Autodesk Fusion 360 part; units mm, degrees
(part 15 of 18)
  arc A2317 (195.6454, -39.5852) -> (195.5255, -39.5852) centre (195.5855, -39.5852) ccw
  arc A2318 (195.5255, -77.7107) -> (195.6454, -77.7107) centre (195.5855, -77.7107) ccw
  arc A2319 (195.6454, -77.7107) -> (195.5255, -77.7107) centre (195.5855, -77.7107) ccw
  arc A2320 (195.5255, -58.648) -> (195.6454, -58.648) centre (195.5855, -58.648) ccw
  arc A2321 (195.6454, -58.648) -> (195.5255, -58.648) centre (195.5855, -58.648) ccw
  arc A2322 (195.6454, -20.5352) -> (195.5255, -20.5352) centre (195.5855, -20.5352) ccw
  arc A2323 (195.5255, -20.5352) -> (195.6454, -20.5352) centre (195.5855, -20.5352) ccw
  arc A2324 (203.2985, -3.41) -> (203.1785, -3.41) centre (203.2385, -3.41) ccw
  arc A2325 (203.1785, -3.41) -> (203.2985, -3.41) centre (203.2385, -3.41) ccw
  arc A2326 (201.3935, -6.331) -> (201.2735, -6.331) centre (201.3335, -6.331) ccw
  arc A2327 (201.2735, -6.331) -> (201.3935, -6.331) centre (201.3335, -6.331) ccw
  arc A2328 (204.8803, -5.2261) -> (205.0003, -5.2261) centre (204.9403, -5.2261) ccw
  arc A2329 (205.0003, -5.2261) -> (204.8803, -5.2261) centre (204.9403, -5.2261) ccw
  arc A2330 (-5.7971, 1.189) -> (-5.6771, 1.189) centre (-5.7371, 1.189) ccw
  arc A2331 (-5.6771, 1.189) -> (-5.7971, 1.189) centre (-5.7371, 1.189) ccw
  arc A2332 (195.2538, -3.4209) -> (195.1338, -3.4209) centre (195.1938, -3.4209) ccw
  arc A2333 (195.1338, -3.4209) -> (195.2538, -3.4209) centre (195.1938, -3.4209) ccw
  arc A2334 (172.1523, -5.568) -> (172.2723, -5.568) centre (172.2123, -5.568) ccw
  arc A2335 (172.2723, -5.568) -> (172.1523, -5.568) centre (172.2123, -5.568) ccw
  arc A2336 (201.4005, -1.505) -> (201.5205, -1.505) centre (201.4605, -1.505) ccw
  arc A2337 (201.5205, -1.505) -> (201.4005, -1.505) centre (201.4605, -1.505) ccw
  arc A2338 (207.5145, -5.263) -> (207.6344, -5.263) centre (207.5744, -5.263) ccw
  arc A2339 (207.6344, -5.263) -> (207.5145, -5.263) centre (207.5744, -5.263) ccw
  arc A2340 (186.8463, -7.1311) -> (186.9662, -7.1311) centre (186.9063, -7.1311) ccw
  arc A2341 (186.9662, -7.1311) -> (186.8463, -7.1311) centre (186.9063, -7.1311) ccw
  arc A2342 (183.8745, -6.331) -> (183.9944, -6.331) centre (183.9345, -6.331) ccw
  arc A2343 (183.9944, -6.331) -> (183.8745, -6.331) centre (183.9345, -6.331) ccw
  arc A2344 (212.5755, -3.786) -> (212.6955, -3.786) centre (212.6355, -3.786) ccw
  arc A2345 (212.6955, -3.786) -> (212.5755, -3.786) centre (212.6355, -3.786) ccw
  arc A2346 (138.4953, -77.7107) -> (138.3754, -77.7107) centre (138.4354, -77.7107) ccw
  arc A2347 (138.3754, -77.7107) -> (138.4953, -77.7107) centre (138.4354, -77.7107) ccw
  arc A2348 (138.3754, -20.5352) -> (138.4953, -20.5352) centre (138.4354, -20.5352) ccw
  arc A2349 (138.4953, -20.5352) -> (138.3754, -20.5352) centre (138.4354, -20.5352) ccw
  arc A2350 (138.3754, -39.5852) -> (138.4953, -39.5852) centre (138.4354, -39.5852) ccw
  arc A2351 (138.4953, -39.5852) -> (138.3754, -39.5852) centre (138.4354, -39.5852) ccw
  arc A2352 (138.4953, -58.648) -> (138.3754, -58.648) centre (138.4354, -58.648) ccw
  arc A2353 (138.3754, -58.648) -> (138.4953, -58.648) centre (138.4354, -58.648) ccw
  arc A2354 (157.5454, -20.5352) -> (157.4254, -20.5352) centre (157.4854, -20.5352) ccw
  arc A2355 (157.4254, -20.5352) -> (157.5454, -20.5352) centre (157.4854, -20.5352) ccw
  arc A2356 (157.5454, -77.7107) -> (157.4254, -77.7107) centre (157.4854, -77.7107) ccw
  arc A2357 (157.4254, -77.7107) -> (157.5454, -77.7107) centre (157.4854, -77.7107) ccw
  arc A2358 (157.4254, -58.648) -> (157.5454, -58.648) centre (157.4854, -58.648) ccw
  arc A2359 (157.5454, -58.648) -> (157.4254, -58.648) centre (157.4854, -58.648) ccw
  arc A2360 (157.4254, -39.5852) -> (157.5454, -39.5852) centre (157.4854, -39.5852) ccw
  arc A2361 (157.5454, -39.5852) -> (157.4254, -39.5852) centre (157.4854, -39.5852) ccw
  arc A2362 (176.4755, -20.5352) -> (176.5954, -20.5352) centre (176.5354, -20.5352) ccw
  arc A2363 (176.5954, -20.5352) -> (176.4755, -20.5352) centre (176.5354, -20.5352) ccw
  arc A2364 (176.5954, -77.7107) -> (176.4755, -77.7107) centre (176.5354, -77.7107) ccw
  arc A2365 (176.4755, -77.7107) -> (176.5954, -77.7107) centre (176.5354, -77.7107) ccw
  arc A2366 (176.4755, -58.648) -> (176.5954, -58.648) centre (176.5354, -58.648) ccw
  arc A2367 (176.5954, -58.648) -> (176.4755, -58.648) centre (176.5354, -58.648) ccw
  arc A2368 (176.4755, -39.5852) -> (176.5954, -39.5852) centre (176.5354, -39.5852) ccw
  arc A2369 (176.5954, -39.5852) -> (176.4755, -39.5852) centre (176.5354, -39.5852) ccw
  arc A2370 (100.3953, -77.7107) -> (100.2753, -77.7107) centre (100.3353, -77.7107) ccw
  arc A2371 (100.2753, -77.7107) -> (100.3953, -77.7107) centre (100.3353, -77.7107) ccw
  arc A2372 (100.3953, -58.648) -> (100.2753, -58.648) centre (100.3353, -58.648) ccw
  arc A2373 (100.2753, -58.648) -> (100.3953, -58.648) centre (100.3353, -58.648) ccw
  arc A2374 (100.3953, -20.5352) -> (100.2753, -20.5352) centre (100.3353, -20.5352) ccw
  arc A2375 (100.2753, -20.5352) -> (100.3953, -20.5352) centre (100.3353, -20.5352) ccw
  arc A2376 (100.3953, -39.5852) -> (100.2753, -39.5852) centre (100.3353, -39.5852) ccw
  arc A2377 (100.2753, -39.5852) -> (100.3953, -39.5852) centre (100.3353, -39.5852) ccw
  arc A2378 (119.4453, -20.5352) -> (119.3253, -20.5352) centre (119.3853, -20.5352) ccw
  arc A2379 (119.3253, -20.5352) -> (119.4453, -20.5352) centre (119.3853, -20.5352) ccw
  arc A2380 (119.3253, -58.648) -> (119.4453, -58.648) centre (119.3853, -58.648) ccw
  arc A2381 (119.4453, -58.648) -> (119.3253, -58.648) centre (119.3853, -58.648) ccw
  arc A2382 (119.3253, -39.5852) -> (119.4453, -39.5852) centre (119.3853, -39.5852) ccw
  arc A2383 (119.4453, -39.5852) -> (119.3253, -39.5852) centre (119.3853, -39.5852) ccw
  arc A2384 (119.3253, -77.7107) -> (119.4453, -77.7107) centre (119.3853, -77.7107) ccw
  arc A2385 (119.4453, -77.7107) -> (119.3253, -77.7107) centre (119.3853, -77.7107) ccw
  arc A2386 (5.0251, -77.7107) -> (5.1451, -77.7107) centre (5.0851, -77.7107) ccw
  arc A2387 (5.1451, -77.7107) -> (5.0251, -77.7107) centre (5.0851, -77.7107) ccw
  arc A2388 (24.0752, -77.7107) -> (24.1951, -77.7107) centre (24.1351, -77.7107) ccw
  arc A2389 (24.1951, -77.7107) -> (24.0752, -77.7107) centre (24.1351, -77.7107) ccw
  arc A2390 (43.1252, -77.7107) -> (43.2451, -77.7107) centre (43.1852, -77.7107) ccw
  arc A2391 (43.2451, -77.7107) -> (43.1252, -77.7107) centre (43.1852, -77.7107) ccw
  arc A2392 (62.2952, -20.5352) -> (62.1752, -20.5352) centre (62.2352, -20.5352) ccw
  arc A2393 (62.1752, -20.5352) -> (62.2952, -20.5352) centre (62.2352, -20.5352) ccw
  arc A2394 (62.1752, -77.7107) -> (62.2952, -77.7107) centre (62.2352, -77.7107) ccw
  arc A2395 (62.2952, -77.7107) -> (62.1752, -77.7107) centre (62.2352, -77.7107) ccw
  arc A2396 (62.1752, -39.5852) -> (62.2952, -39.5852) centre (62.2352, -39.5852) ccw
  arc A2397 (62.2952, -39.5852) -> (62.1752, -39.5852) centre (62.2352, -39.5852) ccw
  arc A2398 (62.1752, -58.648) -> (62.2952, -58.648) centre (62.2352, -58.648) ccw
  arc A2399 (62.2952, -58.648) -> (62.1752, -58.648) centre (62.2352, -58.648) ccw
  arc A2400 (81.2253, -39.5852) -> (81.3452, -39.5852) centre (81.2852, -39.5852) ccw
  arc A2401 (81.3452, -39.5852) -> (81.2253, -39.5852) centre (81.2852, -39.5852) ccw
  arc A2402 (81.2253, -77.7107) -> (81.3452, -77.7107) centre (81.2852, -77.7107) ccw
  arc A2403 (81.3452, -77.7107) -> (81.2253, -77.7107) centre (81.2852, -77.7107) ccw
  arc A2404 (81.2253, -20.5352) -> (81.3452, -20.5352) centre (81.2852, -20.5352) ccw
  arc A2405 (81.3452, -20.5352) -> (81.2253, -20.5352) centre (81.2852, -20.5352) ccw
  arc A2406 (81.3452, -58.648) -> (81.2253, -58.648) centre (81.2852, -58.648) ccw
  arc A2407 (81.2253, -58.648) -> (81.3452, -58.648) centre (81.2852, -58.648) ccw
  arc A2408 (5.0251, -58.648) -> (5.1451, -58.648) centre (5.0851, -58.648) ccw
  arc A2409 (5.1451, -58.648) -> (5.0251, -58.648) centre (5.0851, -58.648) ccw
  arc A2410 (5.0251, -20.5352) -> (5.1451, -20.5352) centre (5.0851, -20.5352) ccw
  arc A2411 (5.1451, -20.5352) -> (5.0251, -20.5352) centre (5.0851, -20.5352) ccw
  arc A2412 (5.1451, -39.5852) -> (5.0251, -39.5852) centre (5.0851, -39.5852) ccw
  arc A2413 (5.0251, -39.5852) -> (5.1451, -39.5852) centre (5.0851, -39.5852) ccw
  arc A2414 (24.0752, -39.5852) -> (24.1951, -39.5852) centre (24.1351, -39.5852) ccw
  arc A2415 (24.1951, -39.5852) -> (24.0752, -39.5852) centre (24.1351, -39.5852) ccw
  arc A2416 (24.0752, -20.5352) -> (24.1951, -20.5352) centre (24.1351, -20.5352) ccw
  arc A2417 (24.1951, -20.5352) -> (24.0752, -20.5352) centre (24.1351, -20.5352) ccw
  arc A2418 (24.0752, -58.648) -> (24.1951, -58.648) centre (24.1351, -58.648) ccw
  arc A2419 (24.1951, -58.648) -> (24.0752, -58.648) centre (24.1351, -58.648) ccw
  arc A2420 (43.1252, -20.5352) -> (43.2451, -20.5352) centre (43.1852, -20.5352) ccw
  arc A2421 (43.2451, -20.5352) -> (43.1252, -20.5352) centre (43.1852, -20.5352) ccw
  arc A2422 (43.1252, -58.648) -> (43.2451, -58.648) centre (43.1852, -58.648) ccw
  arc A2423 (43.2451, -58.648) -> (43.1252, -58.648) centre (43.1852, -58.648) ccw
  arc A2424 (43.2451, -39.5852) -> (43.1252, -39.5852) centre (43.1852, -39.5852) ccw
  arc A2425 (43.1252, -39.5852) -> (43.2451, -39.5852) centre (43.1852, -39.5852) ccw
  arc A2426 (214.6955, -20.5352) -> (214.5755, -20.5352) centre (214.6355, -20.5352) ccw
  arc A2427 (214.5755, -20.5352) -> (214.6955, -20.5352) centre (214.6355, -20.5352) ccw
  arc A2428 (214.6955, -77.7107) -> (214.5755, -77.7107) centre (214.6355, -77.7107) ccw
  arc A2429 (214.5755, -77.7107) -> (214.6955, -77.7107) centre (214.6355, -77.7107) ccw
  arc A2430 (214.5755, -58.648) -> (214.6955, -58.648) centre (214.6355, -58.648) ccw
  arc A2431 (214.6955, -58.648) -> (214.5755, -58.648) centre (214.6355, -58.648) ccw
  arc A2432 (214.6955, -39.5852) -> (214.5755, -39.5852) centre (214.6355, -39.5852) ccw
  arc A2433 (214.5755, -39.5852) -> (214.6955, -39.5852) centre (214.6355, -39.5852) ccw
  arc A2434 (195.5255, -39.5852) -> (195.6454, -39.5852) centre (195.5855, -39.5852) ccw
  arc A2435 (195.6454, -39.5852) -> (195.5255, -39.5852) centre (195.5855, -39.5852) ccw
  arc A2436 (195.6454, -77.7107) -> (195.5255, -77.7107) centre (195.5855, -77.7107) ccw
  arc A2437 (195.5255, -77.7107) -> (195.6454, -77.7107) centre (195.5855, -77.7107) ccw
  arc A2438 (195.6454, -58.648) -> (195.5255, -58.648) centre (195.5855, -58.648) ccw
  arc A2439 (195.5255, -58.648) -> (195.6454, -58.648) centre (195.5855, -58.648) ccw
  arc A2440 (195.5255, -20.5352) -> (195.6454, -20.5352) centre (195.5855, -20.5352) ccw
  arc A2441 (195.6454, -20.5352) -> (195.5255, -20.5352) centre (195.5855, -20.5352) ccw
  arc A2442 (203.2985, -3.41) -> (203.1785, -3.41) centre (203.2385, -3.41) ccw
  arc A2443 (203.1785, -3.41) -> (203.2985, -3.41) centre (203.2385, -3.41) ccw
  arc A2444 (201.3935, -6.331) -> (201.2735, -6.331) centre (201.3335, -6.331) ccw
  arc A2445 (201.2735, -6.331) -> (201.3935, -6.331) centre (201.3335, -6.331) ccw
  arc A2446 (205.0003, -5.2261) -> (204.8803, -5.2261) centre (204.9403, -5.2261) ccw
  arc A2447 (204.8803, -5.2261) -> (205.0003, -5.2261) centre (204.9403, -5.2261) ccw
  arc A2448 (-5.6771, 1.189) -> (-5.7971, 1.189) centre (-5.7371, 1.189) ccw
  arc A2449 (-5.7971, 1.189) -> (-5.6771, 1.189) centre (-5.7371, 1.189) ccw
  arc A2450 (195.2538, -3.4209) -> (195.1338, -3.4209) centre (195.1938, -3.4209) ccw
  arc A2451 (195.1338, -3.4209) -> (195.2538, -3.4209) centre (195.1938, -3.4209) ccw
  arc A2452 (172.1523, -5.568) -> (172.2723, -5.568) centre (172.2123, -5.568) ccw
  arc A2453 (172.2723, -5.568) -> (172.1523, -5.568) centre (172.2123, -5.568) ccw
  arc A2454 (10.2131, -8.0011) -> (9.1131, -8.0011) centre (9.6631, -8.0011) ccw
  arc A2455 (9.1131, -8.0011) -> (10.2131, -8.0011) centre (9.6631, -8.0011) ccw
  arc A2456 (10.2131, -5.4611) -> (9.1131, -5.4611) centre (9.6631, -5.4611) ccw
  arc A2457 (9.1131, -5.4611) -> (10.2131, -5.4611) centre (9.6631, -5.4611) ccw
  arc A2458 (10.2131, -2.9211) -> (9.1131, -2.9211) centre (9.6631, -2.9211) ccw
  arc A2459 (9.1131, -2.9211) -> (10.2131, -2.9211) centre (9.6631, -2.9211) ccw
  arc A2460 (-5.3871, -8.0011) -> (-4.287, -8.0011) centre (-4.8371, -8.0011) ccw
  arc A2461 (-4.287, -8.0011) -> (-5.3871, -8.0011) centre (-4.8371, -8.0011) ccw
  arc A2462 (-4.287, -2.9211) -> (-5.3871, -2.9211) centre (-4.8371, -2.9211) ccw
  arc A2463 (-5.3871, -2.9211) -> (-4.287, -2.9211) centre (-4.8371, -2.9211) ccw
  arc A2464 (175.5224, -4.318) -> (176.5223, -4.318) centre (176.0224, -4.318) ccw
  arc A2465 (176.5223, -4.318) -> (175.5224, -4.318) centre (176.0224, -4.318) ccw
  arc A2466 (173.9823, -4.318) -> (172.9824, -4.318) centre (173.4823, -4.318) ccw
  arc A2467 (172.9824, -4.318) -> (173.9823, -4.318) centre (173.4823, -4.318) ccw
  line L8932 (201.4604, -1.505) -> (201.4604, -2.305)
  line L8933 (201.4604, -2.305) -> (201.1604, -2.305)
  line L8934 (201.1604, -1.505) -> (201.4604, -1.505)
  line L8935 (201.1604, -2.305) -> (201.1604, -1.505)
  line L8936 (199.8604, -1.505) -> (199.8604, -2.305)
  line L8937 (200.1604, -2.305) -> (200.1604, -1.505)
  line L8938 (199.8604, -2.305) -> (200.1604, -2.305)
  line L8939 (200.1604, -1.505) -> (199.8604, -1.505)
  line L8940 (207.5745, -6.0629) -> (207.9745, -6.0629)
  line L8941 (207.9745, -6.2629) -> (207.5745, -6.2629)
  line L8942 (207.5745, -6.2629) -> (207.5745, -6.0629)
  line L8943 (207.9745, -6.0629) -> (207.9745, -6.2629)
  line L8944 (207.9745, -6.6629) -> (207.5745, -6.6629)
  line L8945 (207.9745, -6.4629) -> (207.9745, -6.6629)
  line L8946 (207.5745, -6.6629) -> (207.5745, -6.4629)
  line L8947 (207.5745, -6.4629) -> (207.9745, -6.4629)
  line L8948 (207.9745, -7.0629) -> (207.5745, -7.0629)
  line L8949 (207.9745, -6.8629) -> (207.9745, -7.0629)
  line L8950 (207.5745, -7.0629) -> (207.5745, -6.8629)
  line L8951 (207.5745, -6.8629) -> (207.9745, -6.8629)
  line L8952 (207.9745, -7.4629) -> (207.5745, -7.4629)
  line L8953 (207.5745, -7.2629) -> (207.9745, -7.2629)
  line L8954 (207.5745, -7.4629) -> (207.5745, -7.2629)
  line L8955 (207.9745, -7.2629) -> (207.9745, -7.4629)
  line L8956 (207.5745, -7.6629) -> (207.9745, -7.6629)
  line L8957 (207.9745, -7.6629) -> (207.9745, -7.8629)
  line L8958 (207.5745, -7.8629) -> (207.5745, -7.6629)
  line L8959 (207.9745, -7.8629) -> (207.5745, -7.8629)
  line L8960 (207.5745, -8.0629) -> (207.9745, -8.0629)
  line L8961 (207.9745, -8.2629) -> (207.5745, -8.2629)
  line L8962 (207.9745, -8.0629) -> (207.9745, -8.2629)
  line L8963 (207.5745, -8.2629) -> (207.5745, -8.0629)
  line L8964 (207.9745, -8.4629) -> (207.9745, -8.6629)
  line L8965 (207.5745, -8.4629) -> (207.9745, -8.4629)
  line L8966 (207.9745, -8.6629) -> (207.5745, -8.6629)
  line L8967 (207.5745, -8.6629) -> (207.5745, -8.4629)
  line L8968 (207.5745, -9.0629) -> (207.5745, -8.8629)
  line L8969 (207.9745, -8.8629) -> (207.9745, -9.0629)
  line L8970 (207.5745, -8.8629) -> (207.9745, -8.8629)
  line L8971 (207.9745, -9.0629) -> (207.5745, -9.0629)
  line L8972 (207.9745, -9.2629) -> (207.9745, -9.4629)
  line L8973 (207.5745, -9.2629) -> (207.9745, -9.2629)
  line L8974 (207.5745, -9.4629) -> (207.5745, -9.2629)
  line L8975 (207.9745, -9.4629) -> (207.5745, -9.4629)
  line L8976 (207.9745, -9.6629) -> (207.9745, -9.8629)
  line L8977 (207.5745, -9.8629) -> (207.5745, -9.6629)
  line L8978 (207.9745, -9.8629) -> (207.5745, -9.8629)
  line L8979 (207.5745, -9.6629) -> (207.9745, -9.6629)
  line L8980 (207.5745, -10.2629) -> (207.5745, -10.0629)
  line L8981 (207.5745, -10.0629) -> (207.9745, -10.0629)
  line L8982 (207.9745, -10.2629) -> (207.5745, -10.2629)
  line L8983 (207.9745, -10.0629) -> (207.9745, -10.2629)
  line L8984 (207.5745, -10.6629) -> (207.5745, -10.4629)
  line L8985 (207.9745, -10.4629) -> (207.9745, -10.6629)
  line L8986 (207.9745, -10.6629) -> (207.5745, -10.6629)
  line L8987 (207.5745, -10.4629) -> (207.9745, -10.4629)
  line L8988 (207.9745, -11.0629) -> (207.5745, -11.0629)
  line L8989 (207.5745, -10.8629) -> (207.9745, -10.8629)
  line L8990 (207.9745, -10.8629) -> (207.9745, -11.0629)
  line L8991 (207.5745, -11.0629) -> (207.5745, -10.8629)
  line L8992 (207.9745, -11.4629) -> (207.5745, -11.4629)
  line L8993 (207.5745, -11.4629) -> (207.5745, -11.2629)
  line L8994 (207.9745, -11.2629) -> (207.9745, -11.4629)
  line L8995 (207.5745, -11.2629) -> (207.9745, -11.2629)
  line L8996 (208.5745, -12.2629) -> (208.3745, -12.2629)
  line L8997 (208.3745, -11.8629) -> (208.5745, -11.8629)
  line L8998 (208.3745, -12.2629) -> (208.3745, -11.8629)
  line L8999 (208.5745, -11.8629) -> (208.5745, -12.2629)
  line L9000 (208.9745, -12.2629) -> (208.7745, -12.2629)
  line L9001 (208.9745, -11.8629) -> (208.9745, -12.2629)
  line L9002 (208.7745, -11.8629) -> (208.9745, -11.8629)
  line L9003 (208.7745, -12.2629) -> (208.7745, -11.8629)
  line L9004 (209.1745, -11.8629) -> (209.3745, -11.8629)
  line L9005 (209.3745, -12.2629) -> (209.1745, -12.2629)
  line L9006 (209.1745, -12.2629) -> (209.1745, -11.8629)
  line L9007 (209.3745, -11.8629) -> (209.3745, -12.2629)
  line L9008 (209.5745, -11.8629) -> (209.7745, -11.8629)
  line L9009 (209.7745, -12.2629) -> (209.5745, -12.2629)
  line L9010 (209.7745, -11.8629) -> (209.7745, -12.2629)
  line L9011 (209.5745, -12.2629) -> (209.5745, -11.8629)
  line L9012 (210.1745, -12.2629) -> (209.9745, -12.2629)
  line L9013 (209.9745, -12.2629) -> (209.9745, -11.8629)
  line L9014 (209.9745, -11.8629) -> (210.1745, -11.8629)
  line L9015 (210.1745, -11.8629) -> (210.1745, -12.2629)
  line L9016 (210.3745, -12.2629) -> (210.3745, -11.8629)
  line L9017 (210.5745, -11.8629) -> (210.5745, -12.2629)
  line L9018 (210.5745, -12.2629) -> (210.3745, -12.2629)
  line L9019 (210.3745, -11.8629) -> (210.5745, -11.8629)
  line L9020 (210.7745, -12.2629) -> (210.7745, -11.8629)
  line L9021 (210.9745, -11.8629) -> (210.9745, -12.2629)
  line L9022 (210.7745, -11.8629) -> (210.9745, -11.8629)
  line L9023 (210.9745, -12.2629) -> (210.7745, -12.2629)
  line L9024 (211.3745, -12.2629) -> (211.1745, -12.2629)
  line L9025 (211.1745, -12.2629) -> (211.1745, -11.8629)
  line L9026 (211.3745, -11.8629) -> (211.3745, -12.2629)
  line L9027 (211.1745, -11.8629) -> (211.3745, -11.8629)
  line L9028 (211.7745, -11.8629) -> (211.7745, -12.2629)
  line L9029 (211.5745, -12.2629) -> (211.5745, -11.8629)
  line L9030 (211.7745, -12.2629) -> (211.5745, -12.2629)
  line L9031 (211.5745, -11.8629) -> (211.7745, -11.8629)
  line L9032 (211.9745, -11.8629) -> (212.1745, -11.8629)
  line L9033 (212.1745, -11.8629) -> (212.1745, -12.2629)
  line L9034 (212.1745, -12.2629) -> (211.9745, -12.2629)
  line L9035 (211.9745, -12.2629) -> (211.9745, -11.8629)
  line L9036 (212.3745, -12.2629) -> (212.3745, -11.8629)
  line L9037 (212.5745, -12.2629) -> (212.3745, -12.2629)
  line L9038 (212.3745, -11.8629) -> (212.5745, -11.8629)
  line L9039 (212.5745, -11.8629) -> (212.5745, -12.2629)
  line L9040 (212.7745, -11.8629) -> (212.9745, -11.8629)
  line L9041 (212.7745, -12.2629) -> (212.7745, -11.8629)
  line L9042 (212.9745, -11.8629) -> (212.9745, -12.2629)
  line L9043 (212.9745, -12.2629) -> (212.7745, -12.2629)
  line L9044 (213.3745, -11.8629) -> (213.3745, -12.2629)
  line L9045 (213.1745, -12.2629) -> (213.1745, -11.8629)
  line L9046 (213.3745, -12.2629) -> (213.1745, -12.2629)
  line L9047 (213.1745, -11.8629) -> (213.3745, -11.8629)
  line L9048 (213.7745, -12.2629) -> (213.5745, -12.2629)
  line L9049 (213.5745, -11.8629) -> (213.7745, -11.8629)
  line L9050 (213.5745, -12.2629) -> (213.5745, -11.8629)
  line L9051 (213.7745, -11.8629) -> (213.7745, -12.2629)
  line L9052 (214.5745, -11.4629) -> (214.5745, -11.2629)
  line L9053 (214.1745, -11.2629) -> (214.1745, -11.4629)
  line L9054 (214.5745, -11.2629) -> (214.1745, -11.2629)
  line L9055 (214.1745, -11.4629) -> (214.5745, -11.4629)
  line L9056 (214.5745, -11.0629) -> (214.5745, -10.8629)
  line L9057 (214.1745, -10.8629) -> (214.1745, -11.0629)
  line L9058 (214.5745, -10.8629) -> (214.1745, -10.8629)
  line L9059 (214.1745, -11.0629) -> (214.5745, -11.0629)
  line L9060 (214.1745, -10.6629) -> (214.5745, -10.6629)
  line L9061 (214.5745, -10.6629) -> (214.5745, -10.4629)
  line L9062 (214.1745, -10.4629) -> (214.1745, -10.6629)
  line L9063 (214.5745, -10.4629) -> (214.1745, -10.4629)
  line L9064 (214.5745, -10.2629) -> (214.5745, -10.0629)
  line L9065 (214.1745, -10.2629) -> (214.5745, -10.2629)
  line L9066 (214.5745, -10.0629) -> (214.1745, -10.0629)
  line L9067 (214.1745, -10.0629) -> (214.1745, -10.2629)
  line L9068 (214.1745, -9.8629) -> (214.5745, -9.8629)
  line L9069 (214.5745, -9.6629) -> (214.1745, -9.6629)
  line L9070 (214.5745, -9.8629) -> (214.5745, -9.6629)
  line L9071 (214.1745, -9.6629) -> (214.1745, -9.8629)
  line L9072 (214.5745, -9.4629) -> (214.5745, -9.2629)
  line L9073 (214.1745, -9.2629) -> (214.1745, -9.4629)
  line L9074 (214.1745, -9.4629) -> (214.5745, -9.4629)
  line L9075 (214.5745, -9.2629) -> (214.1745, -9.2629)
  line L9076 (214.5745, -9.0629) -> (214.5745, -8.8629)
  line L9077 (214.1745, -8.8629) -> (214.1745, -9.0629)
  line L9078 (214.1745, -9.0629) -> (214.5745, -9.0629)
  line L9079 (214.5745, -8.8629) -> (214.1745, -8.8629)
  line L9080 (214.1745, -8.4629) -> (214.1745, -8.6629)
  line L9081 (214.5745, -8.4629) -> (214.1745, -8.4629)
  line L9082 (214.5745, -8.6629) -> (214.5745, -8.4629)
  line L9083 (214.1745, -8.6629) -> (214.5745, -8.6629)
  line L9084 (214.1745, -8.2629) -> (214.5745, -8.2629)
  line L9085 (214.1745, -8.0629) -> (214.1745, -8.2629)
  line L9086 (214.5745, -8.2629) -> (214.5745, -8.0629)
  line L9087 (214.5745, -8.0629) -> (214.1745, -8.0629)
  line L9088 (214.1745, -7.8629) -> (214.5745, -7.8629)
  line L9089 (214.5745, -7.6629) -> (214.1745, -7.6629)
  line L9090 (214.1745, -7.6629) -> (214.1745, -7.8629)
  line L9091 (214.5745, -7.8629) -> (214.5745, -7.6629)
  line L9092 (214.5745, -7.4629) -> (214.5745, -7.2629)
  line L9093 (214.5745, -7.2629) -> (214.1745, -7.2629)
  line L9094 (214.1745, -7.4629) -> (214.5745, -7.4629)
  line L9095 (214.1745, -7.2629) -> (214.1745, -7.4629)
  line L9096 (214.1745, -7.0629) -> (214.5745, -7.0629)
  line L9097 (214.5745, -6.8629) -> (214.1745, -6.8629)
  line L9098 (214.5745, -7.0629) -> (214.5745, -6.8629)
  line L9099 (214.1745, -6.8629) -> (214.1745, -7.0629)
  line L9100 (214.5745, -6.6629) -> (214.5745, -6.4629)
  line L9101 (214.1745, -6.6629) -> (214.5745, -6.6629)
  line L9102 (214.1745, -6.4629) -> (214.1745, -6.6629)
  line L9103 (214.5745, -6.4629) -> (214.1745, -6.4629)
  line L9104 (214.1745, -6.2629) -> (214.5745, -6.2629)
  line L9105 (214.5745, -6.0629) -> (214.1745, -6.0629)
  line L9106 (214.5745, -6.2629) -> (214.5745, -6.0629)
  line L9107 (214.1745, -6.0629) -> (214.1745, -6.2629)
  line L9108 (213.7745, -5.6629) -> (213.7745, -5.2629)
  line L9109 (213.5745, -5.2629) -> (213.5745, -5.6629)
  line L9110 (213.7745, -5.2629) -> (213.5745, -5.2629)
  line L9111 (213.5745, -5.6629) -> (213.7745, -5.6629)
  line L9112 (213.3745, -5.2629) -> (213.1745, -5.2629)
  line L9113 (213.3745, -5.6629) -> (213.3745, -5.2629)
  line L9114 (213.1745, -5.2629) -> (213.1745, -5.6629)
  line L9115 (213.1745, -5.6629) -> (213.3745, -5.6629)
  line L9116 (212.7745, -5.6629) -> (212.9745, -5.6629)
  line L9117 (212.9745, -5.2629) -> (212.7745, -5.2629)
  line L9118 (212.9745, -5.6629) -> (212.9745, -5.2629)
  line L9119 (212.7745, -5.2629) -> (212.7745, -5.6629)
  line L9120 (212.3745, -5.2629) -> (212.3745, -5.6629)
  line L9121 (212.5745, -5.6629) -> (212.5745, -5.2629)
  line L9122 (212.5745, -5.2629) -> (212.3745, -5.2629)
  line L9123 (212.3745, -5.6629) -> (212.5745, -5.6629)
  line L9124 (212.1745, -5.6629) -> (212.1745, -5.2629)
  line L9125 (211.9745, -5.2629) -> (211.9745, -5.6629)
  line L9126 (211.9745, -5.6629) -> (212.1745, -5.6629)
  line L9127 (212.1745, -5.2629) -> (211.9745, -5.2629)
  line L9128 (211.7745, -5.6629) -> (211.7745, -5.2629)
  line L9129 (211.7745, -5.2629) -> (211.5745, -5.2629)
  line L9130 (211.5745, -5.6629) -> (211.7745, -5.6629)
  line L9131 (211.5745, -5.2629) -> (211.5745, -5.6629)
  line L9132 (211.3745, -5.2629) -> (211.1745, -5.2629)
  line L9133 (211.3745, -5.6629) -> (211.3745, -5.2629)
  line L9134 (211.1745, -5.6629) -> (211.3745, -5.6629)
  line L9135 (211.1745, -5.2629) -> (211.1745, -5.6629)
  line L9136 (210.9745, -5.2629) -> (210.7745, -5.2629)
  line L9137 (210.7745, -5.2629) -> (210.7745, -5.6629)
  line L9138 (210.9745, -5.6629) -> (210.9745, -5.2629)
  line L9139 (210.7745, -5.6629) -> (210.9745, -5.6629)
  line L9140 (210.5745, -5.6629) -> (210.5745, -5.2629)
  line L9141 (210.3745, -5.6629) -> (210.5745, -5.6629)
  line L9142 (210.5745, -5.2629) -> (210.3745, -5.2629)
  line L9143 (210.3745, -5.2629) -> (210.3745, -5.6629)
  line L9144 (210.1745, -5.6629) -> (210.1745, -5.2629)
  line L9145 (210.1745, -5.2629) -> (209.9745, -5.2629)
  line L9146 (209.9745, -5.6629) -> (210.1745, -5.6629)
  line L9147 (209.9745, -5.2629) -> (209.9745, -5.6629)
  line L9148 (209.7745, -5.6629) -> (209.7745, -5.2629)
  line L9149 (209.5745, -5.2629) -> (209.5745, -5.6629)
  line L9150 (209.7745, -5.2629) -> (209.5745, -5.2629)
  line L9151 (209.5745, -5.6629) -> (209.7745, -5.6629)
  line L9152 (209.3745, -5.6629) -> (209.3745, -5.2629)
  line L9153 (209.3745, -5.2629) -> (209.1745, -5.2629)
  line L9154 (209.1745, -5.2629) -> (209.1745, -5.6629)
  line L9155 (209.1745, -5.6629) -> (209.3745, -5.6629)
  line L9156 (208.7745, -5.6629) -> (208.9745, -5.6629)
  line L9157 (208.7745, -5.2629) -> (208.7745, -5.6629)
  line L9158 (208.9745, -5.2629) -> (208.7745, -5.2629)
  line L9159 (208.9745, -5.6629) -> (208.9745, -5.2629)
  line L9160 (208.5745, -5.6629) -> (208.5745, -5.2629)
  line L9161 (208.3745, -5.6629) -> (208.5745, -5.6629)
  line L9162 (208.5745, -5.2629) -> (208.3745, -5.2629)
  line L9163 (208.3745, -5.2629) -> (208.3745, -5.6629)
  line L9164 (213.0745, -10.7629) -> (209.0745, -10.7629)
  line L9165 (209.0745, -6.7629) -> (213.0745, -6.7629)
  line L9166 (209.0745, -10.7629) -> (209.0745, -6.7629)
  line L9167 (213.0745, -6.7629) -> (213.0745, -10.7629)
  line L9168 (187.2064, -6.331) -> (187.2064, -7.131)
  line L9169 (186.9064, -6.331) -> (187.2064, -6.331)
  line L9170 (187.2064, -7.131) -> (186.9064, -7.131)
  line L9171 (186.9064, -7.131) -> (186.9064, -6.331)
  line L9172 (188.5064, -7.131) -> (188.5064, -6.331)
  line L9173 (188.2064, -7.131) -> (188.5064, -7.131)
  line L9174 (188.2064, -6.331) -> (188.2064, -7.131)
  line L9175 (188.5064, -6.331) -> (188.2064, -6.331)
  line L9176 (183.6344, -7.131) -> (183.6344, -6.331)
  line L9177 (183.9344, -6.331) -> (183.9344, -7.131)
  line L9178 (183.6344, -6.331) -> (183.9344, -6.331)
  line L9179 (183.9344, -7.131) -> (183.6344, -7.131)
  line L9180 (182.6344, -6.331) -> (182.3344, -6.331)
  line L9181 (182.6344, -7.131) -> (182.6344, -6.331)
  line L9182 (182.3344, -6.331) -> (182.3344, -7.131)
  line L9183 (182.3344, -7.131) -> (182.6344, -7.131)
  line L9184 (208.2854, -3.4061) -> (207.7354, -3.4061)
  line L9185 (207.7354, -3.1661) -> (208.2854, -3.1661)
  line L9186 (207.7354, -3.4061) -> (207.7354, -3.1661)
  line L9187 (208.2854, -3.1661) -> (208.2854, -3.4061)
  line L9188 (208.2854, -2.906) -> (207.7354, -2.906)
  line L9189 (207.7354, -2.906) -> (207.7354, -2.666)
  line L9190 (208.2854, -2.666) -> (208.2854, -2.906)
  line L9191 (207.7354, -2.666) -> (208.2854, -2.666)
  line L9192 (207.7354, -2.1659) -> (208.2854, -2.1659)
  line L9193 (208.2854, -2.1659) -> (208.2854, -2.4059)
  line L9194 (208.2854, -2.4059) -> (207.7354, -2.4059)
  line L9195 (207.7354, -2.4059) -> (207.7354, -2.1659)
  line L9196 (207.7354, -1.666) -> (208.2854, -1.666)
  line L9197 (207.7354, -1.906) -> (207.7354, -1.666)
  line L9198 (208.2854, -1.666) -> (208.2854, -1.906)
  line L9199 (208.2854, -1.906) -> (207.7354, -1.906)
  line L9200 (208.2854, -1.4061) -> (207.7354, -1.4061)
  line L9201 (207.7354, -1.4061) -> (207.7354, -1.1661)
  line L9202 (207.7354, -1.1661) -> (208.2854, -1.1661)
  line L9203 (208.2854, -1.1661) -> (208.2854, -1.4061)
  line L9204 (212.0854, -1.1659) -> (212.6354, -1.1659)
  line L9205 (212.6354, -1.4059) -> (212.0854, -1.4059)
  line L9206 (212.6354, -1.1659) -> (212.6354, -1.4059)
  line L9207 (212.0854, -1.4059) -> (212.0854, -1.1659)
  line L9208 (212.0854, -1.666) -> (212.6354, -1.666)
  line L9209 (212.6354, -1.666) -> (212.6354, -1.906)
  line L9210 (212.0854, -1.906) -> (212.0854, -1.666)
  line L9211 (212.6354, -1.906) -> (212.0854, -1.906)
  line L9212 (212.0854, -2.4061) -> (212.0854, -2.1661)
  line L9213 (212.6354, -2.1661) -> (212.6354, -2.4061)
  line L9214 (212.6354, -2.4061) -> (212.0854, -2.4061)
  line L9215 (212.0854, -2.1661) -> (212.6354, -2.1661)
  line L9216 (212.0854, -2.906) -> (212.0854, -2.666)
  line L9217 (212.0854, -2.666) -> (212.6354, -2.666)
  line L9218 (212.6354, -2.906) -> (212.0854, -2.906)
  line L9219 (212.6354, -2.666) -> (212.6354, -2.906)
  line L9220 (212.0854, -3.4059) -> (212.0854, -3.1659)
  line L9221 (212.6354, -3.1659) -> (212.6354, -3.4059)
  line L9222 (212.0854, -3.1659) -> (212.6354, -3.1659)
  line L9223 (212.6354, -3.4059) -> (212.0854, -3.4059)
  line L9224 (138.4353, -76.5606) -> (138.4353, -77.1606)
  line L9225 (138.7853, -77.1606) -> (138.7853, -76.5606)
  line L9226 (138.4353, -77.1606) -> (138.7853, -77.1606)
  line L9227 (138.7853, -76.5606) -> (138.4353, -76.5606)
  line L9228 (142.2353, -77.1606) -> (141.8853, -77.1606)
  line L9229 (141.8853, -77.1606) -> (141.8853, -76.5606)
  line L9230 (142.2353, -76.5606) -> (142.2353, -77.1606)
  line L9231 (141.8853, -76.5606) -> (142.2353, -76.5606)
  line L9232 (138.7853, -19.385) -> (138.4353, -19.385)
  line L9233 (138.7853, -19.985) -> (138.7853, -19.385)
  line L9234 (138.4353, -19.985) -> (138.7853, -19.985)
  line L9235 (138.4353, -19.385) -> (138.4353, -19.985)
  line L9236 (142.2353, -19.985) -> (141.8853, -19.985)
  line L9237 (142.2353, -19.385) -> (142.2353, -19.985)
  line L9238 (141.8853, -19.985) -> (141.8853, -19.385)
  line L9239 (141.8853, -19.385) -> (142.2353, -19.385)
  line L9240 (138.4353, -38.4351) -> (138.4353, -39.0351)
  line L9241 (138.4353, -39.0351) -> (138.7853, -39.0351)
  line L9242 (138.7853, -38.4351) -> (138.4353, -38.4351)
  line L9243 (138.7853, -39.0351) -> (138.7853, -38.4351)
  line L9244 (141.8853, -38.4351) -> (142.2353, -38.4351)
  line L9245 (142.2353, -39.0351) -> (141.8853, -39.0351)
  line L9246 (141.8853, -39.0351) -> (141.8853, -38.4351)
  line L9247 (142.2353, -38.4351) -> (142.2353, -39.0351)
  line L9248 (138.7853, -58.0978) -> (138.7853, -57.4978)
  line L9249 (138.7853, -57.4978) -> (138.4353, -57.4978)
  line L9250 (138.4353, -57.4978) -> (138.4353, -58.0978)
  line L9251 (138.4353, -58.0978) -> (138.7853, -58.0978)
  line L9252 (141.8853, -58.0978) -> (141.8853, -57.4978)
  line L9253 (142.2353, -57.4978) -> (142.2353, -58.0978)
  line L9254 (141.8853, -57.4978) -> (142.2353, -57.4978)
  line L9255 (142.2353, -58.0978) -> (141.8853, -58.0978)
  line L9256 (157.8353, -19.385) -> (157.4853, -19.385)
  line L9257 (157.4853, -19.385) -> (157.4853, -19.985)
  line L9258 (157.4853, -19.985) -> (157.8353, -19.985)
  line L9259 (157.8353, -19.985) -> (157.8353, -19.385)
  line L9260 (160.9353, -19.985) -> (160.9353, -19.385)
  line L9261 (161.2853, -19.385) -> (161.2853, -19.985)
  line L9262 (160.9353, -19.385) -> (161.2853, -19.385)
  line L9263 (161.2853, -19.985) -> (160.9353, -19.985)
  line L9264 (157.8353, -76.5606) -> (157.4853, -76.5606)
  line L9265 (157.8353, -77.1606) -> (157.8353, -76.5606)
  line L9266 (157.4853, -77.1606) -> (157.8353, -77.1606)
  line L9267 (157.4853, -76.5606) -> (157.4853, -77.1606)
  line L9268 (160.9353, -77.1606) -> (160.9353, -76.5606)
  line L9269 (160.9353, -76.5606) -> (161.2853, -76.5606)
  line L9270 (161.2853, -76.5606) -> (161.2853, -77.1606)
  line L9271 (161.2853, -77.1606) -> (160.9353, -77.1606)
  line L9272 (157.4853, -58.0978) -> (157.8353, -58.0978)
  line L9273 (157.8353, -58.0978) -> (157.8353, -57.4978)
  line L9274 (157.8353, -57.4978) -> (157.4853, -57.4978)
  line L9275 (157.4853, -57.4978) -> (157.4853, -58.0978)
  line L9276 (160.9353, -57.4978) -> (161.2853, -57.4978)
  line L9277 (161.2853, -57.4978) -> (161.2853, -58.0978)
  line L9278 (160.9353, -58.0978) -> (160.9353, -57.4978)
  line L9279 (161.2853, -58.0978) -> (160.9353, -58.0978)
  line L9280 (157.4853, -38.4351) -> (157.4853, -39.0351)
  line L9281 (157.8353, -38.4351) -> (157.4853, -38.4351)
  line L9282 (157.8353, -39.0351) -> (157.8353, -38.4351)
  line L9283 (157.4853, -39.0351) -> (157.8353, -39.0351)
  line L9284 (161.2853, -39.0351) -> (160.9353, -39.0351)
  line L9285 (160.9353, -38.4351) -> (161.2853, -38.4351)
  line L9286 (161.2853, -38.4351) -> (161.2853, -39.0351)
  line L9287 (160.9353, -39.0351) -> (160.9353, -38.4351)
  line L9288 (176.5354, -19.985) -> (176.8854, -19.985)
  line L9289 (176.5354, -19.385) -> (176.5354, -19.985)
  line L9290 (176.8854, -19.985) -> (176.8854, -19.385)
  line L9291 (176.8854, -19.385) -> (176.5354, -19.385)
  line L9292 (179.9854, -19.385) -> (180.3354, -19.385)
  line L9293 (179.9854, -19.985) -> (179.9854, -19.385)
  line L9294 (180.3354, -19.385) -> (180.3354, -19.985)
  line L9295 (180.3354, -19.985) -> (179.9854, -19.985)
  line L9296 (176.8854, -77.1606) -> (176.8854, -76.5606)
  line L9297 (176.8854, -76.5606) -> (176.5354, -76.5606)
  line L9298 (176.5354, -77.1606) -> (176.8854, -77.1606)
  line L9299 (176.5354, -76.5606) -> (176.5354, -77.1606)
  line L9300 (179.9854, -76.5606) -> (180.3354, -76.5606)
  line L9301 (180.3354, -76.5606) -> (180.3354, -77.1606)
  line L9302 (179.9854, -77.1606) -> (179.9854, -76.5606)
  line L9303 (180.3354, -77.1606) -> (179.9854, -77.1606)
  line L9304 (176.8854, -58.0978) -> (176.8854, -57.4978)
  line L9305 (176.5354, -57.4978) -> (176.5354, -58.0978)
  line L9306 (176.8854, -57.4978) -> (176.5354, -57.4978)
  line L9307 (176.5354, -58.0978) -> (176.8854, -58.0978)
  line L9308 (179.9854, -58.0978) -> (179.9854, -57.4978)
  line L9309 (180.3354, -58.0978) -> (179.9854, -58.0978)
  line L9310 (179.9854, -57.4978) -> (180.3354, -57.4978)
  line L9311 (180.3354, -57.4978) -> (180.3354, -58.0978)
  line L9312 (176.8854, -39.0351) -> (176.8854, -38.4351)
  line L9313 (176.5354, -39.0351) -> (176.8854, -39.0351)
  line L9314 (176.5354, -38.4351) -> (176.5354, -39.0351)
  line L9315 (176.8854, -38.4351) -> (176.5354, -38.4351)
  line L9316 (180.3354, -39.0351) -> (179.9854, -39.0351)
  line L9317 (180.3354, -38.4351) -> (180.3354, -39.0351)
  line L9318 (179.9854, -38.4351) -> (180.3354, -38.4351)
  line L9319 (179.9854, -39.0351) -> (179.9854, -38.4351)
  line L9320 (100.3352, -77.1606) -> (100.6852, -77.1606)
  line L9321 (100.3352, -76.5606) -> (100.3352, -77.1606)
  line L9322 (100.6852, -76.5606) -> (100.3352, -76.5606)
  line L9323 (100.6852, -77.1606) -> (100.6852, -76.5606)
  line L9324 (104.1352, -77.1606) -> (103.7852, -77.1606)
  line L9325 (104.1352, -76.5606) -> (104.1352, -77.1606)
  line L9326 (103.7852, -77.1606) -> (103.7852, -76.5606)
  line L9327 (103.7852, -76.5606) -> (104.1352, -76.5606)
  line L9328 (100.6852, -57.4978) -> (100.3352, -57.4978)
  line L9329 (100.3352, -58.0978) -> (100.6852, -58.0978)
  line L9330 (100.6852, -58.0978) -> (100.6852, -57.4978)
  line L9331 (100.3352, -57.4978) -> (100.3352, -58.0978)
  line L9332 (104.1352, -58.0978) -> (103.7852, -58.0978)
  line L9333 (104.1352, -57.4978) -> (104.1352, -58.0978)
  line L9334 (103.7852, -58.0978) -> (103.7852, -57.4978)
  line L9335 (103.7852, -57.4978) -> (104.1352, -57.4978)
  line L9336 (100.6852, -19.985) -> (100.6852, -19.385)
  line L9337 (100.3352, -19.385) -> (100.3352, -19.985)
  line L9338 (100.3352, -19.985) -> (100.6852, -19.985)
  line L9339 (100.6852, -19.385) -> (100.3352, -19.385)
  line L9340 (104.1352, -19.385) -> (104.1352, -19.985)
  line L9341 (103.7852, -19.385) -> (104.1352, -19.385)
  line L9342 (104.1352, -19.985) -> (103.7852, -19.985)
  line L9343 (103.7852, -19.985) -> (103.7852, -19.385)
  line L9344 (100.6852, -38.4351) -> (100.3352, -38.4351)
  line L9345 (100.6852, -39.0351) -> (100.6852, -38.4351)
  line L9346 (100.3352, -38.4351) -> (100.3352, -39.0351)
  line L9347 (100.3352, -39.0351) -> (100.6852, -39.0351)
  line L9348 (104.1352, -39.0351) -> (103.7852, -39.0351)
  line L9349 (103.7852, -39.0351) -> (103.7852, -38.4351)
  line L9350 (103.7852, -38.4351) -> (104.1352, -38.4351)
  line L9351 (104.1352, -38.4351) -> (104.1352, -39.0351)
  line L9352 (119.7352, -19.985) -> (119.7352, -19.385)
  line L9353 (119.3852, -19.985) -> (119.7352, -19.985)
  line L9354 (119.7352, -19.385) -> (119.3852, -19.385)
  line L9355 (119.3852, -19.385) -> (119.3852, -19.985)
  line L9356 (123.1852, -19.985) -> (122.8352, -19.985)
  line L9357 (122.8352, -19.385) -> (123.1852, -19.385)
  line L9358 (122.8352, -19.985) -> (122.8352, -19.385)
  line L9359 (123.1852, -19.385) -> (123.1852, -19.985)
  line L9360 (119.3852, -58.0978) -> (119.7352, -58.0978)
  line L9361 (119.3852, -57.4978) -> (119.3852, -58.0978)
  line L9362 (119.7352, -57.4978) -> (119.3852, -57.4978)
  line L9363 (119.7352, -58.0978) -> (119.7352, -57.4978)
  line L9364 (123.1852, -57.4978) -> (123.1852, -58.0978)
  line L9365 (122.8352, -57.4978) -> (123.1852, -57.4978)
  line L9366 (122.8352, -58.0978) -> (122.8352, -57.4978)
  line L9367 (123.1852, -58.0978) -> (122.8352, -58.0978)
  line L9368 (119.7352, -38.4351) -> (119.3852, -38.4351)
  line L9369 (119.3852, -38.4351) -> (119.3852, -39.0351)
  line L9370 (119.3852, -39.0351) -> (119.7352, -39.0351)
  line L9371 (119.7352, -39.0351) -> (119.7352, -38.4351)
  line L9372 (123.1852, -38.4351) -> (123.1852, -39.0351)
  line L9373 (123.1852, -39.0351) -> (122.8352, -39.0351)
  line L9374 (122.8352, -38.4351) -> (123.1852, -38.4351)
  line L9375 (122.8352, -39.0351) -> (122.8352, -38.4351)
  line L9376 (119.7352, -77.1606) -> (119.7352, -76.5606)
  line L9377 (119.7352, -76.5606) -> (119.3852, -76.5606)
  line L9378 (119.3852, -76.5606) -> (119.3852, -77.1606)
  line L9379 (119.3852, -77.1606) -> (119.7352, -77.1606)
  line L9380 (122.8352, -76.5606) -> (123.1852, -76.5606)
  line L9381 (123.1852, -77.1606) -> (122.8352, -77.1606)
  line L9382 (122.8352, -77.1606) -> (122.8352, -76.5606)
  line L9383 (123.1852, -76.5606) -> (123.1852, -77.1606)
  line L9384 (5.435, -76.5606) -> (5.085, -76.5606)
  line L9385 (5.435, -77.1606) -> (5.435, -76.5606)
  line L9386 (5.085, -76.5606) -> (5.085, -77.1606)
  line L9387 (5.085, -77.1606) -> (5.435, -77.1606)
  line L9388 (8.535, -76.5606) -> (8.885, -76.5606)
  line L9389 (8.885, -76.5606) -> (8.885, -77.1606)
  line L9390 (8.535, -77.1606) -> (8.535, -76.5606)
  line L9391 (8.885, -77.1606) -> (8.535, -77.1606)
  line L9392 (24.4851, -76.5606) -> (24.1351, -76.5606)
  line L9393 (24.1351, -76.5606) -> (24.1351, -77.1606)
  line L9394 (24.1351, -77.1606) -> (24.4851, -77.1606)
  line L9395 (24.4851, -77.1606) -> (24.4851, -76.5606)
  line L9396 (27.5851, -76.5606) -> (27.9351, -76.5606)
  line L9397 (27.9351, -77.1606) -> (27.5851, -77.1606)
  line L9398 (27.5851, -77.1606) -> (27.5851, -76.5606)
  line L9399 (27.9351, -76.5606) -> (27.9351, -77.1606)
  line L9400 (43.1851, -77.1606) -> (43.5351, -77.1606)
  line L9401 (43.5351, -77.1606) -> (43.5351, -76.5606)
  line L9402 (43.1851, -76.5606) -> (43.1851, -77.1606)
  line L9403 (43.5351, -76.5606) -> (43.1851, -76.5606)
  line L9404 (46.6351, -76.5606) -> (46.9851, -76.5606)
  line L9405 (46.9851, -77.1606) -> (46.6351, -77.1606)
  line L9406 (46.6351, -77.1606) -> (46.6351, -76.5606)
  line L9407 (46.9851, -76.5606) -> (46.9851, -77.1606)
  line L9408 (62.2351, -19.985) -> (62.5851, -19.985)
  line L9409 (62.5851, -19.385) -> (62.2351, -19.385)
  line L9410 (62.2351, -19.385) -> (62.2351, -19.985)
  line L9411 (62.5851, -19.985) -> (62.5851, -19.385)
  line L9412 (66.0351, -19.985) -> (65.6851, -19.985)
  line L9413 (65.6851, -19.985) -> (65.6851, -19.385)
  line L9414 (66.0351, -19.385) -> (66.0351, -19.985)
  line L9415 (65.6851, -19.385) -> (66.0351, -19.385)
  line L9416 (62.5851, -76.5606) -> (62.2351, -76.5606)
  line L9417 (62.5851, -77.1606) -> (62.5851, -76.5606)
  line L9418 (62.2351, -76.5606) -> (62.2351, -77.1606)
  line L9419 (62.2351, -77.1606) -> (62.5851, -77.1606)
  line L9420 (65.6851, -77.1606) -> (65.6851, -76.5606)
  line L9421 (66.0351, -76.5606) -> (66.0351, -77.1606)
  line L9422 (65.6851, -76.5606) -> (66.0351, -76.5606)
  line L9423 (66.0351, -77.1606) -> (65.6851, -77.1606)
  line L9424 (62.2351, -39.0351) -> (62.5851, -39.0351)
  line L9425 (62.5851, -39.0351) -> (62.5851, -38.4351)
  line L9426 (62.2351, -38.4351) -> (62.2351, -39.0351)
  line L9427 (62.5851, -38.4351) -> (62.2351, -38.4351)
  line L9428 (65.6851, -39.0351) -> (65.6851, -38.4351)
  line L9429 (66.0351, -38.4351) -> (66.0351, -39.0351)
  line L9430 (65.6851, -38.4351) -> (66.0351, -38.4351)
  line L9431 (66.0351, -39.0351) -> (65.6851, -39.0351)
  line L9432 (62.5851, -57.4978) -> (62.2351, -57.4978)
  line L9433 (62.5851, -58.0978) -> (62.5851, -57.4978)
  line L9434 (62.2351, -58.0978) -> (62.5851, -58.0978)
  line L9435 (62.2351, -57.4978) -> (62.2351, -58.0978)
  line L9436 (65.6851, -58.0978) -> (65.6851, -57.4978)
  line L9437 (65.6851, -57.4978) -> (66.0351, -57.4978)
  line L9438 (66.0351, -58.0978) -> (65.6851, -58.0978)
  line L9439 (66.0351, -57.4978) -> (66.0351, -58.0978)
  line L9440 (81.2852, -38.4351) -> (81.2852, -39.0351)
  line L9441 (81.2852, -39.0351) -> (81.6352, -39.0351)
  line L9442 (81.6352, -38.4351) -> (81.2852, -38.4351)
  line L9443 (81.6352, -39.0351) -> (81.6352, -38.4351)
  line L9444 (84.7352, -39.0351) -> (84.7352, -38.4351)
  line L9445 (85.0852, -39.0351) -> (84.7352, -39.0351)
  line L9446 (84.7352, -38.4351) -> (85.0852, -38.4351)
  line L9447 (85.0852, -38.4351) -> (85.0852, -39.0351)
  line L9448 (81.2852, -77.1606) -> (81.6352, -77.1606)
  line L9449 (81.6352, -76.5606) -> (81.2852, -76.5606)
  line L9450 (81.6352, -77.1606) -> (81.6352, -76.5606)
  line L9451 (81.2852, -76.5606) -> (81.2852, -77.1606)
  line L9452 (84.7352, -77.1606) -> (84.7352, -76.5606)
  line L9453 (85.0852, -76.5606) -> (85.0852, -77.1606)
  line L9454 (84.7352, -76.5606) -> (85.0852, -76.5606)
  line L9455 (85.0852, -77.1606) -> (84.7352, -77.1606)
  line L9456 (81.6352, -19.385) -> (81.2852, -19.385)
  line L9457 (81.2852, -19.985) -> (81.6352, -19.985)
  line L9458 (81.6352, -19.985) -> (81.6352, -19.385)
  line L9459 (81.2852, -19.385) -> (81.2852, -19.985)
  line L9460 (84.7352, -19.985) -> (84.7352, -19.385)
  line L9461 (85.0852, -19.985) -> (84.7352, -19.985)
  line L9462 (85.0852, -19.385) -> (85.0852, -19.985)
  line L9463 (84.7352, -19.385) -> (85.0852, -19.385)
  line L9464 (81.6352, -57.4978) -> (81.2852, -57.4978)
  line L9465 (81.2852, -58.0978) -> (81.6352, -58.0978)
  line L9466 (81.2852, -57.4978) -> (81.2852, -58.0978)
  line L9467 (81.6352, -58.0978) -> (81.6352, -57.4978)
  line L9468 (84.7352, -58.0978) -> (84.7352, -57.4978)
  line L9469 (85.0852, -58.0978) -> (84.7352, -58.0978)
  line L9470 (85.0852, -57.4978) -> (85.0852, -58.0978)
  line L9471 (84.7352, -57.4978) -> (85.0852, -57.4978)
  line L9472 (5.435, -58.0978) -> (5.435, -57.4978)
  line L9473 (5.085, -58.0978) -> (5.435, -58.0978)
  line L9474 (5.435, -57.4978) -> (5.085, -57.4978)
  line L9475 (5.085, -57.4978) -> (5.085, -58.0978)
  line L9476 (8.535, -58.0978) -> (8.535, -57.4978)
  line L9477 (8.885, -58.0978) -> (8.535, -58.0978)
  line L9478 (8.885, -57.4978) -> (8.885, -58.0978)
  line L9479 (8.535, -57.4978) -> (8.885, -57.4978)
  line L9480 (5.085, -19.985) -> (5.435, -19.985)
  line L9481 (5.435, -19.385) -> (5.085, -19.385)
  line L9482 (5.435, -19.985) -> (5.435, -19.385)
  line L9483 (5.085, -19.385) -> (5.085, -19.985)
  line L9484 (8.885, -19.985) -> (8.535, -19.985)
  line L9485 (8.535, -19.985) -> (8.535, -19.385)
  line L9486 (8.535, -19.385) -> (8.885, -19.385)
  line L9487 (8.885, -19.385) -> (8.885, -19.985)
  line L9488 (5.435, -39.0351) -> (5.435, -38.4351)
  line L9489 (5.085, -39.0351) -> (5.435, -39.0351)
  line L9490 (5.435, -38.4351) -> (5.085, -38.4351)
  line L9491 (5.085, -38.4351) -> (5.085, -39.0351)
  line L9492 (8.535, -38.4351) -> (8.885, -38.4351)
  line L9493 (8.535, -39.0351) -> (8.535, -38.4351)
  line L9494 (8.885, -39.0351) -> (8.535, -39.0351)
  line L9495 (8.885, -38.4351) -> (8.885, -39.0351)
  line L9496 (24.1351, -39.0351) -> (24.4851, -39.0351)
  line L9497 (24.4851, -39.0351) -> (24.4851, -38.4351)
  line L9498 (24.4851, -38.4351) -> (24.1351, -38.4351)
  line L9499 (24.1351, -38.4351) -> (24.1351, -39.0351)
  line L9500 (27.5851, -39.0351) -> (27.5851, -38.4351)
  line L9501 (27.9351, -38.4351) -> (27.9351, -39.0351)
  line L9502 (27.5851, -38.4351) -> (27.9351, -38.4351)
  line L9503 (27.9351, -39.0351) -> (27.5851, -39.0351)
  line L9504 (24.4851, -19.985) -> (24.4851, -19.385)
  line L9505 (24.1351, -19.985) -> (24.4851, -19.985)
  line L9506 (24.4851, -19.385) -> (24.1351, -19.385)
  line L9507 (24.1351, -19.385) -> (24.1351, -19.985)
  line L9508 (27.9351, -19.985) -> (27.5851, -19.985)
  line L9509 (27.5851, -19.985) -> (27.5851, -19.385)
  line L9510 (27.5851, -19.385) -> (27.9351, -19.385)
  line L9511 (27.9351, -19.385) -> (27.9351, -19.985)
  line L9512 (24.1351, -58.0978) -> (24.4851, -58.0978)
  line L9513 (24.4851, -58.0978) -> (24.4851, -57.4978)
  line L9514 (24.4851, -57.4978) -> (24.1351, -57.4978)
  line L9515 (24.1351, -57.4978) -> (24.1351, -58.0978)
  line L9516 (27.5851, -57.4978) -> (27.9351, -57.4978)
  line L9517 (27.9351, -58.0978) -> (27.5851, -58.0978)
  line L9518 (27.5851, -58.0978) -> (27.5851, -57.4978)
  line L9519 (27.9351, -57.4978) -> (27.9351, -58.0978)
  line L9520 (43.5351, -19.385) -> (43.1851, -19.385)
  line L9521 (43.1851, -19.385) -> (43.1851, -19.985)
  line L9522 (43.1851, -19.985) -> (43.5351, -19.985)
  line L9523 (43.5351, -19.985) -> (43.5351, -19.385)
  line L9524 (46.9851, -19.385) -> (46.9851, -19.985)
  line L9525 (46.6351, -19.385) -> (46.9851, -19.385)
  line L9526 (46.6351, -19.985) -> (46.6351, -19.385)
  line L9527 (46.9851, -19.985) -> (46.6351, -19.985)
  line L9528 (43.1851, -57.4978) -> (43.1851, -58.0978)
  line L9529 (43.5351, -57.4978) -> (43.1851, -57.4978)
  line L9530 (43.5351, -58.0978) -> (43.5351, -57.4978)
  line L9531 (43.1851, -58.0978) -> (43.5351, -58.0978)
  line L9532 (46.9851, -58.0978) -> (46.6351, -58.0978)
  line L9533 (46.6351, -57.4978) -> (46.9851, -57.4978)
  line L9534 (46.6351, -58.0978) -> (46.6351, -57.4978)
  line L9535 (46.9851, -57.4978) -> (46.9851, -58.0978)
  line L9536 (43.1851, -38.4351) -> (43.1851, -39.0351)
  line L9537 (43.1851, -39.0351) -> (43.5351, -39.0351)
  line L9538 (43.5351, -38.4351) -> (43.1851, -38.4351)
  line L9539 (43.5351, -39.0351) -> (43.5351, -38.4351)
  line L9540 (46.9851, -39.0351) -> (46.6351, -39.0351)
  line L9541 (46.6351, -38.4351) -> (46.9851, -38.4351)
  line L9542 (46.9851, -38.4351) -> (46.9851, -39.0351)
  line L9543 (46.6351, -39.0351) -> (46.6351, -38.4351)
  line L9544 (214.9854, -19.985) -> (214.9854, -19.385)
  line L9545 (214.6354, -19.985) -> (214.9854, -19.985)
  line L9546 (214.9854, -19.385) -> (214.6354, -19.385)
  line L9547 (214.6354, -19.385) -> (214.6354, -19.985)
  line L9548 (218.4354, -19.385) -> (218.4354, -19.985)
  line L9549 (218.0854, -19.385) -> (218.4354, -19.385)
  line L9550 (218.4354, -19.985) -> (218.0854, -19.985)
  line L9551 (218.0854, -19.985) -> (218.0854, -19.385)
  line L9552 (214.9854, -77.1606) -> (214.9854, -76.5606)
  line L9553 (214.9854, -76.5606) -> (214.6354, -76.5606)
  line L9554 (214.6354, -77.1606) -> (214.9854, -77.1606)
  line L9555 (214.6354, -76.5606) -> (214.6354, -77.1606)
  line L9556 (218.4354, -76.5606) -> (218.4354, -77.1606)
  line L9557 (218.0854, -76.5606) -> (218.4354, -76.5606)
  line L9558 (218.0854, -77.1606) -> (218.0854, -76.5606)
  line L9559 (218.4354, -77.1606) -> (218.0854, -77.1606)
  line L9560 (214.9854, -58.0978) -> (214.9854, -57.4978)
  line L9561 (214.9854, -57.4978) -> (214.6354, -57.4978)
  line L9562 (214.6354, -57.4978) -> (214.6354, -58.0978)
  line L9563 (214.6354, -58.0978) -> (214.9854, -58.0978)
  line L9564 (218.4354, -57.4978) -> (218.4354, -58.0978)
  line L9565 (218.0854, -58.0978) -> (218.0854, -57.4978)
  line L9566 (218.0854, -57.4978) -> (218.4354, -57.4978)
  line L9567 (218.4354, -58.0978) -> (218.0854, -58.0978)
  line L9568 (214.6354, -38.4351) -> (214.6354, -39.0351)
  line L9569 (214.9854, -39.0351) -> (214.9854, -38.4351)
  line L9570 (214.6354, -39.0351) -> (214.9854, -39.0351)
  line L9571 (214.9854, -38.4351) -> (214.6354, -38.4351)
  line L9572 (218.0854, -39.0351) -> (218.0854, -38.4351)
  line L9573 (218.4354, -39.0351) -> (218.0854, -39.0351)
  line L9574 (218.4354, -38.4351) -> (218.4354, -39.0351)
  line L9575 (218.0854, -38.4351) -> (218.4354, -38.4351)
  line L9576 (195.9354, -38.4351) -> (195.5854, -38.4351)
  line L9577 (195.9354, -39.0351) -> (195.9354, -38.4351)
  line L9578 (195.5854, -39.0351) -> (195.9354, -39.0351)
  line L9579 (195.5854, -38.4351) -> (195.5854, -39.0351)
  line L9580 (199.0354, -39.0351) -> (199.0354, -38.4351)
  line L9581 (199.0354, -38.4351) -> (199.3854, -38.4351)
  line L9582 (199.3854, -38.4351) -> (199.3854, -39.0351)
  line L9583 (199.3854, -39.0351) -> (199.0354, -39.0351)
  line L9584 (195.5854, -76.5606) -> (195.5854, -77.1606)
  line L9585 (195.5854, -77.1606) -> (195.9354, -77.1606)
  line L9586 (195.9354, -77.1606) -> (195.9354, -76.5606)
  line L9587 (195.9354, -76.5606) -> (195.5854, -76.5606)
  line L9588 (199.3854, -76.5606) -> (199.3854, -77.1606)